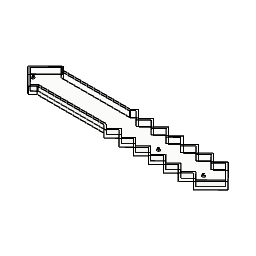
Enclosure (Autodesk Fusion 360 archive; units mm, degrees)
design "Top"
Autodesk Fusion 360 part; units mm, degrees
sketch "Skeleton" plane through (0, 0, 0) normal (0, 0, 1) x (1, 0, 0)
  line L0 (277.5, 0) -> (256.2938, -20.8843)
  line L1 (256.2938, -20.8843) -> (246.2384, -10.674)
  line L2 (256.6758, 21.1455) -> (246.2384, 10.8666)
  line L3 (235.8638, 21.4001) -> (246.2384, 10.8666)
  line L4 (235.8638, 21.4001) -> (224.9913, 10.6915)
  line L5 (235.4726, -21.3127) -> (224.9913, -10.7061)
  line L6 (224.9913, -10.7061) -> (214.1025, -21.4307)
  line L7 (214.1025, -21.4307) -> (203.4049, -10.5694)
  line L8 (203.4049, 10.4421) -> (192.8642, 21.1442)
  line L9 (192.8642, 21.1442) -> (182.3597, 10.7981)
  line L10 (214.4868, 21.3569) -> (203.4049, 10.4421)
  line L11 (214.4868, 21.3569) -> (224.9913, 10.6915)
  line L12 (246.2384, -10.674) -> (235.4726, -21.3127)
  line L13 (150.6753, 21.4115) -> (160.9404, 10.9892)
  line L14 (192.5671, -21.2437) -> (182.3597, -10.88)
  line L15 (171.7172, 21.6035) -> (160.9404, 10.9892)
  line L16 (171.7172, 21.6035) -> (182.3597, 10.7981)
  line L17 (203.4049, -10.5694) -> (192.5671, -21.2437)
  line L18 (128.5744, 22.0844) -> (139.7933, 10.6936)
  line L19 (160.9404, -10.9256) -> (171.4645, -21.6108)
  line L20 (123.723, -15.3938) -> (128.859, -20.6084)
  line L21 (22.1658, 21.8316) -> (26.623, 17.3062)
  line L22 (11.6354, 11.46) -> (0, 0)
  line L23 (0, 0) -> (20.8053, -21.1238)
  line L24 (20.8053, -21.1238) -> (26.623, -15.3938)
  line L25 (11.6354, 11.46) -> (22.1658, 21.8316)
  line L26 (128.5744, 22.0844) -> (123.723, 17.3062)
  line L27 (139.7933, -9.839) -> (128.859, -20.6084)
  line L28 (160.9404, -10.9256) -> (150.7494, -20.9628)
  line L29 (150.6753, 21.4115) -> (139.7933, 10.6936)
  line L30 (182.3597, -10.88) -> (171.4645, -21.6108)
  line L31 (150.7494, -20.9628) -> (139.7933, -9.839)
  line L32 (277.5, 0) -> (0, 0) construction
  line L33 (26.623, 17.3062) -> (123.723, 17.3062)
  line L34 (26.623, -15.3938) -> (123.723, -15.3938)
  line L35 (26.623, 17.3062) -> (26.623, -15.3938) construction
  line L36 (123.723, 17.3062) -> (123.723, -15.3938) construction
  line L37 (277.5, 0) -> (256.6758, 21.1455)
  line L38 (139.7933, 10.6936) -> (139.7933, -9.839) construction
  line L39 (160.9404, 10.9892) -> (160.9404, -10.9256) construction
  line L40 (182.3597, -10.88) -> (182.3597, 10.7981) construction
  line L41 (203.4049, -10.5694) -> (203.4049, 10.4421) construction
  line L42 (224.9913, -10.7061) -> (224.9913, 10.6915) construction
  line L43 (246.2384, 10.8666) -> (246.2384, -10.674) construction
  line L44 (281.0615, 0.3027) -> (256.1148, -24.2653)
  line L45 (256.1148, -24.2653) -> (245.8517, -13.8441)
  line L46 (245.8517, -13.8441) -> (234.9999, -24.5678)
  line L47 (234.9999, -24.5678) -> (224.8789, -14.3258)
  line L48 (224.8789, -14.3258) -> (214.0756, -24.9662)
  line L49 (214.0756, -24.9662) -> (203.378, -14.1048)
  line L50 (203.378, -14.1048) -> (192.5402, -24.7792)
  line L51 (192.5402, -24.7792) -> (182.3328, -14.4154)
  line L52 (182.3328, -14.4154) -> (171.5048, -25.0801)
  line L53 (160.9807, -14.3948) -> (171.5048, -25.0801)
  line L54 (160.9807, -14.3948) -> (150.7296, -24.4914)
  line L55 (150.7296, -24.4914) -> (139.7735, -13.3675)
  line L56 (139.7735, -13.3675) -> (128.8321, -24.1439)
  line L57 (122.6763, -17.8938) -> (128.8321, -24.1439)
  line L58 (27.6474, -17.8938) -> (122.6763, -17.8938)
  line L59 (20.7784, -24.6593) -> (27.6474, -17.8938)
  line L60 (-3.5354, 0.0269) -> (20.7784, -24.6593)
  line L61 (9.8812, 13.2411) -> (-3.5354, 0.0269)
  line L62 (9.8812, 13.2411) -> (22.1927, 25.367)
  line L63 (22.1927, 25.367) -> (27.6697, 19.8062)
  line L64 (27.6697, 19.8062) -> (122.6986, 19.8062)
  line L65 (128.5943, 25.6129) -> (122.6986, 19.8062)
  line L66 (128.5943, 25.6129) -> (139.8064, 14.2291)
  line L67 (150.6344, 24.8937) -> (139.8064, 14.2291)
  line L68 (150.6344, 24.8937) -> (160.9063, 14.4646)
  line L69 (171.7441, 25.1389) -> (160.9063, 14.4646)
  line L70 (171.7441, 25.1389) -> (182.7002, 14.0151)
  line L71 (193.508, 24.6599) -> (182.7002, 14.0151)
  line L72 (204.0322, 13.9746) -> (193.508, 24.6599)
  line L73 (214.9142, 24.6926) -> (204.0322, 13.9746)
  line L74 (214.9142, 24.6926) -> (225.1216, 14.3289)
  line L75 (235.8907, 24.9355) -> (225.1216, 14.3289)
  line L76 (235.8907, 24.9355) -> (246.5883, 14.0741)
  line L77 (257.2038, 24.5284) -> (246.5883, 14.0741)
  line L78 (281.0615, 0.3027) -> (257.2038, 24.5284)
  arc A0 (4.912, -4.9872) -> (4.9872, 4.912) centre (0, 0) ccw
  circle A1 centre (4, 0) radius 1
  circle A2 centre (182.3597, -0.041) radius 2.5
  circle A3 centre (246.2384, 0.0963) radius 2.5
  circle A4 centre (182.3597, -0.041) radius 1
  circle A5 centre (246.2384, 0.0963) radius 1
  dimension "d1" = 32.7
  dimension "d2" = 97.1
  dimension "d15" = 7
  dimension "d16" = 2
  dimension "d17" = 4
  dimension "d18" = 5
  dimension "d19" = 5
  dimension "d20" = 2
  dimension "d21" = 2
  constraint parallel L20 L31
  constraint parallel L14 L19
  constraint parallel L7 L14
  constraint coincident L23.end L24.start
  constraint coincident L22.end L23.start
  constraint coincident L22.start L25.start
  constraint coincident L21.start L25.end
  constraint perpendicular L20 L27
  constraint coincident L20.end L27.end
  constraint coincident L27.start L31.end
  constraint coincident L18.start L26.start
  constraint perpendicular L28 L31
  constraint coincident L28.end L31.start
  constraint coincident L19.start L28.start
  constraint coincident L13.start L29.start
  constraint coincident L19.end L30.end
  constraint perpendicular L19 L30
  constraint perpendicular L14 L17
  constraint coincident L14.end L30.start
  constraint coincident L15.start L16.start
  constraint perpendicular L6 L7
  constraint coincident L14.start L17.end
  constraint perpendicular L5 L12
  constraint perpendicular L0 L1
  constraint coincident L6.end L7.start
  constraint coincident L3.start L4.start
  constraint coincident L2.end L3.end
  constraint coincident L0.end L1.start
  constraint horizontal L33
  constraint horizontal L34
  constraint vertical L35
  constraint vertical L36
  constraint perpendicular L2 L37
  constraint coincident L13.end L15.end
  constraint coincident L1.end L12.start
  constraint coincident L22 A0.end
  constraint coincident L32 A1.centre
  constraint parallel L0 L44
  constraint parallel L1 L45
  constraint parallel L12 L46
  constraint parallel L5 L47
  constraint parallel L6 L48
  constraint parallel L7 L49
  constraint parallel L17 L50
  constraint parallel L14 L51
  constraint parallel L30 L52
  constraint parallel L19 L53
  constraint parallel L28 L54
  constraint parallel L31 L55
  constraint parallel L27 L56
  constraint parallel L20 L57
  constraint parallel L34 L58
  constraint parallel L24 L59
  constraint parallel L23 L60
  constraint parallel L22 L61
  constraint parallel L25 L62
  constraint parallel L21 L63
  constraint parallel L33 L64
  constraint parallel L26 L65
  constraint parallel L18 L66
  constraint parallel L29 L67
  constraint parallel L13 L68
  constraint parallel L15 L69
  constraint parallel L16 L70
  constraint parallel L9 L71
  constraint parallel L8 L72
  constraint parallel L10 L73
  constraint parallel L11 L74
  constraint parallel L4 L75
  constraint parallel L3 L76
  constraint parallel L2 L77
  constraint parallel L37 L78
  constraint vertical L43
  constraint vertical L42
  constraint vertical L41
  constraint vertical L40
  constraint vertical L39
  constraint vertical L38
  constraint midpoint L40 A2.centre
  constraint midpoint L43 A3.centre
  constraint concentric A2 A4
  constraint concentric A3 A5
  measures "d1" distance of L21.end L24.end
  measures "d2" distance of L21.end L26.end
  measures "d15" radius of A0
  measures "d16" diameter of A1
  measures "d17" horizontal distance of L22.end A1.centre
  measures "d18" diameter of A2
  measures "d19" diameter of A3
  measures "d20" diameter of A4
  measures "d21" diameter of A5
extrude "Extrude1" add sketch "Skeleton" along normal blind 8 contours L44 L45 L46 L47 L48 L49 L50 L51 L52 L53 L54 L55 L56 L57 L58 L59 L60 L61 L62 L63 L64 L65 L66 L67 L68 L69 L70 L71 L72 L73 L74 L75 L76 L77 L78
extrude "Extrude2" add sketch "Skeleton" against normal blind 2.5 contours L0 L1 L2 L3 L4 L5 L6 L7 L8 L9 L10 L11 L12 L13 L14 L15 L16 L17 L18 L19 L20 L21 L22 L23 L24 L25 L26 L27 L28 L29 L30 L31 L33 L34 L37 A0 | L22 L23 A0 | L44 L45 L46 L47 L48 L49 L50 L51 L52 L53 L54 L55 L56 L57 L58 L59 L60 L61 L62 L63 L64 L65 L66 L67 L68 L69 L70 L71 L72 L73 L74 L75 L76 L77 L78 | A1 | A2 | A3 | A4 | A5
fillet "Fillet1" radius 1.25 2 edges at (22.1927, 25.367, 2.75) (20.7784, -24.6593, 2.75)
extrude "Extrude7" cut sketch "Skeleton" against normal up to surface (2.5 mm away) contours A1 | A4 | A5
chamfer "Chamfer2" distance 1 angle 45 3 edges at (245.3061, -0.2653, -2.5) (181.4273, -0.4026, -2.5) (3.0677, -0.3616, -2.5)
equation "wall_thickness = 2.5 mm"
equation "d5 = height"
equation "height = 8 mm"
equation "d8 = -wall_thickness"
equation "d11 = wall_thickness / 2"
equation "d24 = 45 mm - 2 mm - 2 mm"
equation "d25 = 30 mm - 2 mm - 2 mm"
equation "d26 = 30 mm - 2 mm - 2 mm"
equation "d27 = 25 mm - 2 mm - 2 mm"
